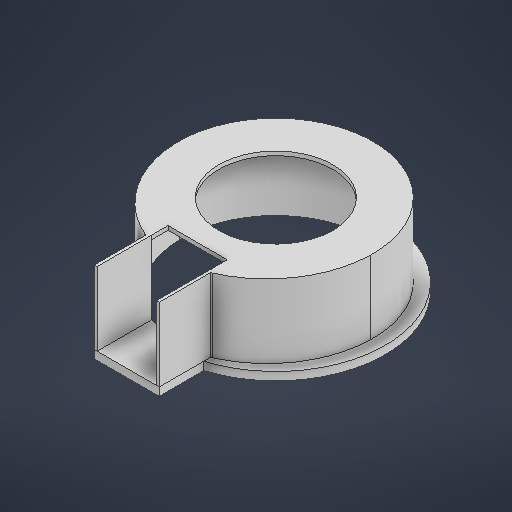
# Autodesk Inventor part: Cylinder Housing Optical Camera
Saved by Autodesk Inventor 2025 (Build 290162000, 162)
## iProperties
Created: 2025-08-14
Part Number: Cylinder Housing Optical Camera
Material: Generic
Document SubType Name: Modeling
Designer: mayhem
Density: 1 g/cm^3
Appearance: Default
Author: mayhem
Autodesk Inventor part; units mm, degrees
ref_plane "YZ Plane" through (0, 0, 0) normal (1, 0, 0) x (0, 1, 0)
ref_plane "XZ Plane" through (0, 0, 0) normal (0, 1, 0) x (-1, 0, 0)
ref_plane "XY Plane" through (0, 0, 0) normal (0, 0, 1) x (1, 0, 0)
sketch "Sketch1" plane through (0, 0, 0) normal (0, 1, 0) x (-1, 0, 0)
  arc A0 (-40.0043, 128.9366) -> (39.9957, 128.9393) centre (0, 0) ccw
  line L0 (-40.0043, 128.9366) -> (-40.0043, 183.9366)
  line L1 (-40.0043, 183.9366) -> (39.9957, 183.9393)
  line L2 (39.9957, 183.9393) -> (39.9957, 128.9393)
  arc A1 (-114.9519, 3.3257) -> (114.9519, 3.3257) centre (0, 0) ccw
  arc A2 (114.9519, 3.3257) -> (39.9957, 115.0039) centre (-11.1576, -0.3228) ccw
  line L3 (0, -135) -> (0, -115)
  arc A3 (-39.9957, 115.0039) -> (-114.9519, 3.3257) centre (11.1576, -0.3228) ccw
  arc A4 (39.9957, 115.0039) -> (-39.9957, 115.0039) centre (0, 24.8323) ccw
  point P0 (0, 128.7652)
  point P1 (-0.0043, -3.5634)
  point P2 (-0.0043, 183.938)
  dimension "d0" = 270
  dimension "d7" = 80
  dimension "d9" = 230
  dimension "d13" = 55
  dimension "d26" = 55
  constraints: 14 point on circle, 8 end point, 5 centre point, 3 tangent, 2 coincident, 2 symmetric about line, 1 midpoint, 1 parallel, 1 vertical, 1 other
  measures "d0" diameter of A0
  measures "d7" distance of L0.end L1.end
  measures "d9" diameter of A1
  measures "d13" distance of L0.start L0.end
  measures "d26" distance of L1.end L2.end
extrude "Extrusion1" add sketch "Sketch1" along normal blind 10
sketch "Sketch5" plane through (0, 10, 0) normal (0, 1, 0) x (1, 0, 0)
  arc A0 (114.9519, -3.3257) -> (-114.9519, -3.3257) centre (0, 0) ccw projected
  arc A1 (-114.9519, -3.3257) -> (-39.9957, -115.0039) centre (11.1576, 0.3228) ccw projected
  arc A2 (-39.9957, -115.0039) -> (39.9957, -115.0039) centre (0, -24.8323) ccw projected
  arc A3 (39.9957, -115.0039) -> (114.9519, -3.3257) centre (-11.1576, 0.3228) ccw projected
  arc A4 (119.9498, -3.4703) -> (-119.9498, -3.4703) centre (0, 0) ccw
  arc A5 (42.023, -119.5745) -> (119.9498, -3.4703) centre (-11.1576, 0.3228) ccw
  arc A6 (-119.9498, -3.4703) -> (-42.023, -119.5745) centre (11.1576, 0.3228) ccw
  line L0 (-39.9957, -183.9393) -> (40.0043, -183.9366) projected
  line L1 (-39.9957, -183.9366) -> (-39.9957, -120.448)
  line L2 (40.0043, -120.4444) -> (40.0043, -183.9366)
  line L3 (-36.4957, -116.4764) -> (-36.4957, -183.9366)
  line L4 (36.5043, -183.9366) -> (36.5043, -116.473)
  arc A7 (-42.023, -119.5745) -> (-39.9957, -120.448) centre (0, -24.8323) ccw
  arc A8 (40.0043, -120.4444) -> (42.023, -119.5745) centre (0, -24.8323) ccw
  line L5 (40.0043, -183.9366) -> (36.5043, -183.9366)
  line L6 (-36.4957, -183.9366) -> (-39.9957, -183.9366)
  dimension "d24" = 5
  dimension "d27" = 3.5
  constraints: 12 end point, 12 point on circle, 5 centre point, 2 horizontal, 2 parallel, 2 perpendicular, 1 other
  measures "d24" radial gap between concentric circles of A0 A4
  measures "d27" distance between parallel lines of L1 L3
extrude "Extrusion3" add sketch "Sketch5" along normal blind 90.5 contours A0 A1 A2 L3 L6 L1 A7 A6 A4 A5 A8 L2 L0 L4 A3
sketch "Sketch6" plane through (0, 100.5, 0) normal (0, 1, 0) x (1, 0, 0)
  arc A0 (114.9519, -3.3257) -> (-114.9519, -3.3257) centre (0, 0) ccw projected
  arc A1 (-114.9519, -3.3257) -> (-39.9957, -115.0039) centre (11.1576, 0.3228) ccw projected
  arc A2 (-36.4957, -116.4764) -> (36.5043, -116.473) centre (0, -24.8323) ccw projected
  arc A3 (39.9957, -115.0039) -> (114.9519, -3.3257) centre (-11.1576, 0.3228) ccw projected
  arc A4 (36.5043, -116.473) -> (39.9957, -115.0039) centre (0, -24.8323) ccw projected
  arc A5 (-39.9957, -115.0039) -> (-36.4957, -116.4764) centre (0, -24.8323) ccw projected
  circle A6 centre (0, 0) radius 70.375
  line L0 (-36.4957, -116.4764) -> (-36.4967, -96.4764)
  line L1 (-36.4967, -96.4764) -> (36.5033, -96.473)
  line L2 (36.5033, -96.473) -> (36.5043, -116.473)
  dimension "d30" = 140.75
  dimension "d33" = 20
  constraints: 6 end point, 1 centre point, 1 coincident, 1 parallel
  measures "d30" diameter of A6
  measures "d33" distance of L0.start L0.end
extrude "Extrusion4" add sketch "Sketch6" against normal blind 5 contours A3 A4 L2 L1 L0 A5 A1 A0
body "Solid1"
